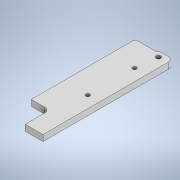
# Autodesk Inventor part: Upper slide
Saved by Autodesk Inventor 2021 (Build 250183000, 183)
## iProperties
Created: 2020-08-14
Part Number: Upper slide
Material: Generic
Document SubType Name: Modeling
Designer: jgray
Density: 1 g/cm^3
Appearance: Default
Author: jgray
Autodesk Inventor part; units mm, degrees
ref_plane "YZ Plane" through (0, 0, 0) normal (1, 0, 0) x (0, 1, 0)
ref_plane "XZ Plane" through (0, 0, 0) normal (0, 1, 0) x (-1, 0, 0)
ref_plane "XY Plane" through (0, 0, 0) normal (0, 0, 1) x (1, 0, 0)
sketch "Sketch1" plane through (0, 0, 0) normal (0, 1, 0) x (-1, 0, 0)
  line L0 (0, 0) -> (29.5, 0)
  line L1 (29.5, -15) -> (29.5, -102.5)
  line L2 (0.8775, -104.5) -> (0, -104.5)
  line L3 (0, -102.5) -> (0, -15)
  line L4 (0, -93.5) -> (0, -102)
  line L5 (0, -43.5) -> (0, -56.5)
  line L6 (29.5, 0) -> (0, 0)
  line L7 (0, 0) -> (0, -15)
  line L8 (29.5, -15) -> (29.5, 0)
  arc A0 (27.5, -104.5) -> (29.5, -102.5) centre (27.5, -102.5) ccw
  line L9 (27.5, -104.5) -> (12, -104.5)
  line L10 (27.5, -104.5) -> (12, -104.5)
  line L11 (0, -104.5) -> (0.8775, -104.5)
  line L12 (12, -104.5) -> (12, -106)
  line L13 (12, -106) -> (4, -106)
  line L14 (0, -102) -> (0, -104.5)
  arc A1 (0, -102) -> (4, -106) centre (4, -102) ccw
  point P0 (29.5, -104.5)
  point P1 (11, -104.5)
  point P2 (0, -102)
  point P3 (0, -106)
  dimension "d0" = 29.5
  dimension "d1" = 104.5
  dimension "d7" = 15
  dimension "d8" = 2
  dimension "d40" = 12
  dimension "d41" = 1.5
  dimension "d42" = 4
  constraints: 31 end point, 9 point on line, 5 horizontal, 5 parallel, 5 point on circle, 4 tangent, 3 perpendicular, 2 centre point, 1 collinear
  measures "d0" distance of point (29.5, -104.5) L2.end
  measures "d1" distance of L0.end point (29.5, -104.5)
  measures "d7" distance of L3.end L6.end
  measures "d8" radius of A0
  measures "d40" distance of L12.end point (0, -106)
  measures "d41" distance of L9.end L12.end
  measures "d42" radius of A1
extrude "Extrusion1" add sketch "Sketch1" along normal blind 5 contours L0 L8 L1 A0 L9 L12 L13 A1 L3 L7
sketch "Sketch2" plane through (0, 5, 0) normal (0, 1, 0) x (1, 0, 0)
  line L0 (-9.5, -6.918) -> (-9.5, 116.4057) construction
  line L1 (0, 0) -> (0, 102) construction
  line L2 (-29.5, 102.5) -> (-29.5, 0) projected
  point P0 (-9.5, 84)
  point P1 (-9.5, 46)
  point P2 (-29.5, 16)
  point P3 (0, 16)
  point P4 (0, 102.5)
  point P5 (0, 104.5)
  dimension "d13" = 46
  dimension "d14" = 84
  dimension "d23" = 20
  constraints: 2 end point, 2 point on line, 1 vertical
  measures "d13" vertical distance of point (-9.5, 46) L1.start
  measures "d14" vertical distance of L1.start point (-9.5, 84)
  measures "d23" distance between parallel lines of L2 L0
hole "Hole1" at (-9.5, 5, -84) at (-9.5, 5, -46) direction (0, -1, 0) diameter 3.2 end through all
sketch "Sketch3" plane through (0, 5, 0) normal (0, 1, 0) x (1, 0, 0)
  line L0 (-29.5, 0) -> (0, 0) projected
  line L1 (-29.5, 0) -> (-14.5, 0)
  line L2 (-14.5, 0) -> (-14.5, 16)
  line L3 (-18.5, 20) -> (-29.5, 20)
  line L4 (-29.5, 20) -> (-29.5, 0)
  arc A0 (-14.5, 16) -> (-18.5, 20) centre (-18.5, 16) ccw
  point P0 (-14.5, 20)
  dimension "d26" = 15
  dimension "d27" = 20
  dimension "d28" = 4
  constraints: 8 end point, 2 parallel, 2 point on circle, 2 point on line, 2 tangent, 1 centre point, 1 horizontal, 1 perpendicular
  measures "d26" distance of L3.end point (-14.5, 20)
  measures "d27" distance of point (-14.5, 20) L1.end
  measures "d28" radius of A0
extrude "Extrusion2" cut sketch "Sketch3" against normal through all
sketch "Sketch4" plane through (0, 5, 0) normal (0, 1, 0) x (1, 0, 0)
  line L0 (0, 0) -> (0, 102) projected
  line L1 (-4, 106) -> (-12, 106) projected
  point P0 (-7.5, 101.5)
  dimension "d31" = 7.5
  dimension "d43" = 4.5
  measures "d31" distance from line of L0 point (-7.5, 101.5)
  measures "d43" distance from line of point (-7.5, 101.5) L1
hole "Hole2" at (-7.5, 5, -101.5) direction (0, -1, 0) diameter 3.8 end through all
fillet "Fillet1" radius 2 1 edges at (-12, 2.5, -106)
body "Solid1"
